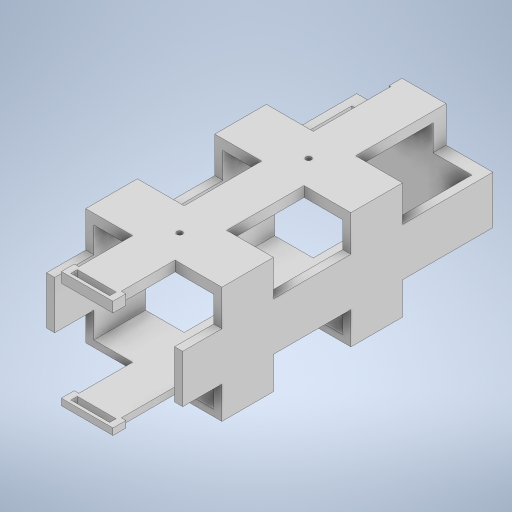
# Autodesk Inventor part: battery holder v2
Saved by Autodesk Inventor 2023 (Build 270158000, 158)
## iProperties
Created: 2023-01-11
Part Number: battery holder v2
Material: Generic
Document SubType Name: Modeling
Designer: agent
Density: 1 g/cm^3
Appearance: Default
Author: agent
Autodesk Inventor part; units mm, degrees
ref_plane "YZ Plane" through (0, 0, 0) normal (1, 0, 0) x (0, 1, 0)
ref_plane "XZ Plane" through (0, 0, 0) normal (0, 1, 0) x (-1, 0, 0)
ref_plane "XY Plane" through (0, 0, 0) normal (0, 0, 1) x (1, 0, 0)
sketch "Sketch1" plane through (0, 0, 0) normal (0, 1, 0) x (-1, 0, 0)
  line L0 (125.7746, -116.0471) -> (66.7746, -116.0471)
  line L1 (66.7746, -116.0471) -> (66.7746, 37.4129)
  line L2 (66.7746, 37.4129) -> (125.7746, 37.4129)
  line L3 (125.7746, 37.4129) -> (125.7746, -116.0471)
  point P0 (0, 0)
  dimension "d0" = 59
  dimension "d1" = 153.46
  constraints: 8 end point, 2 parallel, 1 horizontal, 1 perpendicular
  measures "d0" distance of L1.end L2.end
  measures "d1" distance between parallel lines of L2 L0
extrude "Extrusion1" add sketch "Sketch1" along normal blind 49
sketch "Sketch2" plane through (0, 0, 0) normal (0, -1, 0) x (1, 0, 0)
  line L0 (-125.7746, 37.4129) -> (-66.7746, 37.4129) projected
  line L1 (-66.7746, -116.0471) -> (-125.7746, -116.0471) projected
  line L2 (-85.8246, 37.4129) -> (-106.7246, 37.4129)
  line L3 (-106.7246, 37.4129) -> (-106.7246, -116.0471)
  line L4 (-106.7246, -116.0471) -> (-85.8246, -116.0471)
  line L5 (-85.8246, -116.0471) -> (-85.8246, 37.4129)
  line L6 (-66.7746, 37.4129) -> (-66.7746, -116.0471) projected
  line L7 (-125.7746, -116.0471) -> (-125.7746, 37.4129) projected
  point P0 (0, 0)
  dimension "d4" = 19.05
  dimension "d5" = 19.05
  constraints: 8 end point, 2 parallel, 2 point on line, 1 horizontal, 1 perpendicular
  measures "d4" distance between parallel lines of L6 L5
  measures "d5" distance between parallel lines of L7 L3
extrude "Extrusion2" add sketch "Sketch2" along normal blind 3.22 contours L0 L5 L1 L3
sketch "Sketch3" plane through (0, 49, 0) normal (0, 1, 0) x (1, 0, 0)
  line L0 (-125.7746, -37.4129) -> (-66.7746, -37.4129) projected
  line L1 (-106.7246, 116.0471) -> (-125.7746, 116.0471) projected
  line L2 (-85.8246, -37.4129) -> (-106.7246, -37.4129)
  line L3 (-106.7246, -37.4129) -> (-106.7246, 116.0471)
  line L4 (-106.7246, 116.0471) -> (-85.8246, 116.0471)
  line L5 (-85.8246, 116.0471) -> (-85.8246, -37.4129)
  line L6 (-66.7746, -37.4129) -> (-66.7746, 116.0471) projected
  line L7 (-125.7746, 116.0471) -> (-125.7746, -37.4129) projected
  point P0 (0, 0)
  dimension "d8" = 19.05
  dimension "d9" = 19.05
  constraints: 8 end point, 2 parallel, 2 point on line, 1 horizontal, 1 perpendicular
  measures "d8" distance between parallel lines of L6 L5
  measures "d9" distance between parallel lines of L7 L3
extrude "Extrusion3" add sketch "Sketch3" along normal blind 5 contours L3 L4 L5 L0
sketch "Sketch4" plane through (-66.7746, 0, 37.4129) normal (1, 0, 0) x (0, 0, -1)
  line L0 (0, 0) -> (0, 49) projected
  line L1 (153.46, 0) -> (153.46, 49) projected
  line L2 (0, 36.3) -> (153.46, 36.3)
  line L3 (153.46, 36.3) -> (153.46, 12.7)
  line L4 (153.46, 12.7) -> (0, 12.7)
  line L5 (0, 12.7) -> (0, 36.3)
  line L6 (0, 49) -> (153.46, 49) projected
  line L7 (0, 0) -> (153.46, 0) projected
  point P0 (37.4129, 0)
  point P1 (0, 12.7)
  dimension "d12" = 12.7
  dimension "d13" = 12.7
  constraints: 8 end point, 2 parallel, 2 point on line, 1 horizontal, 1 perpendicular
  measures "d12" distance between parallel lines of L6 L2
  measures "d13" distance between parallel lines of L7 L4
extrude "Extrusion4" add sketch "Sketch4" along normal blind 4 contours L0 L2 L1 L4
sketch "Sketch5" plane through (-125.7746, 0, -116.0471) normal (-1, 0, 0) x (0, 0, 1)
  line L0 (153.46, 0) -> (153.46, 49) projected
  line L1 (0, 0) -> (0, 49) projected
  line L2 (153.46, 12.7) -> (0, 12.7)
  line L3 (0, 12.7) -> (0, 36.3)
  line L4 (0, 36.3) -> (153.46, 36.3)
  line L5 (153.46, 36.3) -> (153.46, 12.7)
  line L6 (0, 0) -> (153.46, 0) projected
  line L7 (0, 49) -> (153.46, 49) projected
  point P0 (116.0471, 0)
  point P1 (0, 12.7)
  dimension "d16" = 12.7
  dimension "d17" = 12.7
  constraints: 8 end point, 2 parallel, 2 point on line, 1 horizontal, 1 perpendicular
  measures "d16" distance between parallel lines of L6 L2
  measures "d17" distance between parallel lines of L7 L4
extrude "Extrusion5" add sketch "Sketch5" along normal blind 4 contours L2 L1 L4 L0
sketch "Sketch6" plane through (-66.7746, 0, -116.0471) normal (0, 0, -1) x (-1, 0, 0)
  line L0 (63, -3.22) -> (-4, -3.22)
  line L1 (-4, -3.22) -> (-4, 54)
  line L2 (-4, 54) -> (63, 54)
  line L3 (63, 54) -> (63, -3.22)
  line L4 (19.05, 54) -> (39.95, 54) projected
  line L5 (63, 36.3) -> (63, 12.7) projected
  line L6 (-4, 12.7) -> (-4, 36.3) projected
  point P0 (-66.7746, 0)
  dimension "d20" = 0
  dimension "d21" = 0
  dimension "d22" = 0
  constraints: 8 end point, 2 parallel, 1 horizontal, 1 perpendicular
  measures "d20" distance between parallel lines of L4 L2
  measures "d21" distance between parallel lines of L5 L3
  measures "d22" distance between parallel lines of L6 L1
extrude "Extrusion6" add sketch "Sketch6" along normal blind 6.395
sketch "Sketch7" plane through (-129.7746, 0, -116.0471) normal (-1, 0, 0) x (0, 0, 1)
  line L0 (153.46, 54) -> (0, 54) projected
  line L1 (153.46, -3.22) -> (0, -3.22) projected
  line L2 (38.1, 54) -> (63.5, 54)
  line L3 (63.5, 54) -> (63.5, -3.22)
  line L4 (63.5, -3.22) -> (38.1, -3.22)
  line L5 (38.1, -3.22) -> (38.1, 54)
  line L6 (101.6, 54) -> (127, 54)
  line L7 (127, 54) -> (127, -3.22)
  line L8 (127, -3.22) -> (101.6, -3.22)
  line L9 (101.6, -3.22) -> (101.6, 54)
  line L10 (0, 36.3) -> (0, 54) projected
  point P0 (116.0471, 0)
  point P1 (127, -3.22)
  dimension "d25" = 38.1
  dimension "d26" = 38.1
  dimension "d27" = 25.4
  dimension "d28" = 25.4
  constraints: 16 end point, 4 parallel, 4 point on line, 2 horizontal, 2 perpendicular
  measures "d25" distance between parallel lines of L10 L5
  measures "d26" distance between parallel lines of L9 L3
  measures "d27" distance between parallel lines of L3 L5
  measures "d28" distance between parallel lines of L7 L9
extrude "Extrusion7" add sketch "Sketch7" against normal up to surface (67 mm away) contours L7 L1 L9 L0 | L3 L1 L5 L0
sketch "Sketch8" plane through (-125.7746, 0, 37.4129) normal (0, 0, 1) x (1, 0, 0)
  line L0 (39.95, 49) -> (59, 49) projected
  line L1 (-4, 54) -> (19.05, 54) projected
  line L2 (42.2021, 49) -> (16.8021, 49)
  line L3 (16.8021, 49) -> (16.8021, 54)
  line L4 (16.8021, 54) -> (42.2021, 54)
  line L5 (42.2021, 54) -> (42.2021, 49)
  line L6 (19.05, 49) -> (19.05, 54) projected
  line L7 (0, 0) -> (19.05, 0) projected
  line L8 (39.95, -3.22) -> (63, -3.22) projected
  line L9 (16.8021, 0) -> (42.2021, 0)
  line L10 (42.2021, 0) -> (42.2021, -3.22)
  line L11 (42.2021, -3.22) -> (16.8021, -3.22)
  line L12 (16.8021, -3.22) -> (16.8021, 0)
  point P0 (125.7746, 0)
  point P1 (42.2021, 51.5)
  point P2 (16.8021, 51.5)
  point P3 (19.05, 51.5)
  dimension "d31" = 25.4
  dimension "d32" = 2.2479
  constraints: 16 end point, 4 parallel, 4 point on line, 3 midpoint, 2 horizontal, 2 perpendicular
  measures "d31" distance of point (42.202, 51.5) point (16.802, 51.5)
  measures "d32" distance of point (16.802, 51.5) point (19.05, 51.5)
extrude "Extrusion8" add sketch "Sketch8" along normal blind 6.35
sketch "Sketch9" plane through (0, 54, 0) normal (0, 1, 0) x (1, 0, 0)
  line L0 (-118.2456, -83.2824) -> (-137.2956, -83.2824)
  line L1 (-137.2956, -83.2824) -> (-137.2956, -80.1074)
  line L2 (-137.2956, -80.1074) -> (-118.2456, -80.1074)
  line L3 (-118.2456, -80.1074) -> (-118.2456, -83.2824)
  line L4 (-86.7475, -39.0639) -> (-105.7975, -39.0639)
  line L5 (-105.7975, -39.0639) -> (-105.7975, -42.2389)
  line L6 (-105.7975, -42.2389) -> (-86.7475, -42.2389)
  line L7 (-86.7475, -42.2389) -> (-86.7475, -39.0639)
  line L8 (-83.5725, -43.7629) -> (-108.9725, -43.7629) projected
  line L9 (-83.5725, -37.4129) -> (-83.5725, -43.7629) projected
  point P0 (0, 0)
  point P1 (-118.2456, -81.6949)
  point P2 (-137.2956, -81.6949)
  point P3 (-105.7975, -40.6514)
  point P4 (-86.7475, -40.6514)
  point P5 (-83.5725, -40.5879)
  dimension "d35" = 3.175
  dimension "d36" = 19.05
  dimension "d37" = 19.05
  dimension "d38" = 3.175
  dimension "d39" = 1.524
  dimension "d40" = 3.175
  constraints: 16 end point, 5 midpoint, 3 parallel, 1 horizontal, 1 perpendicular
  measures "d35" distance between parallel lines of L0 L2
  measures "d36" distance of point (-118.246, -81.695) point (-137.296, -81.695)
  measures "d37" distance from line of point (-105.797, -40.651) L7
  measures "d38" distance between parallel lines of L4 L6
  measures "d39" distance between parallel lines of L8 L6
  measures "d40" horizontal distance of point (-86.747, -40.651) point (-83.572, -40.588)
extrude "Extrusion9" cut sketch "Sketch9" against normal up to surface (57.22 mm away) contours L7 L6 L5 L4
sketch "Sketch10" plane through (-66.7746, 12.7, 37.4129) normal (0, 0, 1) x (1, 0, 0)
  line L0 (-59, 23.6) -> (-59, 36.3) projected
  line L1 (0, 0) -> (0, -12.7) projected
  line L2 (-59, 36.3) -> (0, 36.3)
  line L3 (0, 36.3) -> (0, -12.7)
  line L4 (0, -12.7) -> (-59, -12.7)
  line L5 (-59, -12.7) -> (-59, 36.3)
  point P0 (66.7746, -12.7)
  point P1 (-59, 23.6)
  constraints: 8 end point, 2 parallel, 1 horizontal, 1 perpendicular
extrude "Extrusion10" cut sketch "Sketch10" against normal up to surface (153.46 mm away)
sketch "Sketch11" plane through (0, 54, 0) normal (0, 1, 0) x (1, 0, 0)
  line L0 (-85.8246, 116.0471) -> (-85.8246, 77.9471) projected
  line L1 (-129.7746, 52.5471) -> (-106.7246, 52.5471) projected
  line L2 (-85.8246, 52.5471) -> (-85.8246, 14.4471) projected
  line L3 (-129.7746, -10.9529) -> (-106.7246, -10.9529) projected
  circle A0 centre (-96.2746, 65.2471) radius 1.35
  circle A1 centre (-96.2746, 1.7471) radius 1.35
  point P0 (0, 0)
  dimension "d45" = 2.7
  dimension "d46" = 2.7
  dimension "d47" = 63.5
  constraints: 2 centre point
  measures "d45" diameter of A0
  measures "d46" diameter of A1
  measures "d47" distance of A1.centre A0.centre
extrude "Extrusion11" cut sketch "Sketch11" against normal up to surface (57.22 mm away)
sketch "Sketch12" plane through (-108.9725, 49, 43.7629) normal (0, -1, 0) x (1, 0, 0)
  circle A0 centre (12.6979, -45.51) radius 1.35 projected
  circle A1 centre (12.6979, -45.51) radius 3.175
  circle A2 centre (12.6979, -109.01) radius 1.35 projected
  circle A3 centre (12.6979, -109.01) radius 3.175
  point P0 (108.9725, -43.7629)
  dimension "d50" = 6.35
  dimension "d51" = 6.35
  constraints: 2 centre point, 2 coincident
  measures "d50" diameter of A1
  measures "d51" diameter of A3
extrude "Extrusion12" cut sketch "Sketch12" against normal blind 2 contours A0 | A1 | A2 | A3
sketch "Sketch13" plane through (-129.7746, 0, -116.0471) normal (-1, 0, 0) x (0, 0, 1)
  line L0 (153.46, 36.3) -> (127, 36.3) projected
  line L1 (127, 12.7) -> (153.46, 12.7) projected
  line L2 (153.46, 36.3) -> (146.2804, 36.3)
  line L3 (146.2804, 36.3) -> (146.2804, 12.7)
  line L4 (146.2804, 12.7) -> (153.46, 12.7)
  line L5 (153.46, 12.7) -> (153.46, 36.3)
  point P0 (116.0471, 0)
  constraints: 8 end point, 2 parallel, 1 horizontal, 1 perpendicular, 1 point on line
extrude "Extrusion13" cut sketch "Sketch13" against normal up to surface (67 mm away)
sketch "Sketch14" plane through (-66.7746, 0, -122.4421) normal (0, 0, -1) x (-1, 0, 0)
  line L0 (-4, 36.3) -> (-4, 54) projected
  line L1 (-4, 54) -> (19.05, 54)
  line L2 (19.05, 54) -> (19.05, 36.3)
  line L3 (19.05, 36.3) -> (-4, 36.3)
  line L4 (-4, 36.3) -> (-4, 54)
  line L5 (63, -3.22) -> (63, 54) projected
  line L6 (63, 54) -> (40.73, 54)
  line L7 (40.73, 54) -> (40.73, 36.3)
  line L8 (40.73, 36.3) -> (63, 36.3)
  line L9 (63, 36.3) -> (63, 54)
  line L10 (63, 12.7) -> (63, -3.22) projected
  line L11 (63, -3.22) -> (39.95, -3.22) projected
  line L12 (63, 12.7) -> (39.95, 12.7)
  line L13 (39.95, 12.7) -> (39.95, -3.22)
  line L14 (39.95, -3.22) -> (63, -3.22)
  line L15 (63, -3.22) -> (63, 12.7)
  line L16 (-4, 12.7) -> (-4, -3.22) projected
  line L17 (-4, -3.22) -> (19.05, -3.22)
  line L18 (19.05, -3.22) -> (19.05, 12.7)
  line L19 (19.05, 12.7) -> (-4, 12.7)
  line L20 (-4, 12.7) -> (-4, -3.22)
  point P0 (-66.7746, 0)
  point P1 (19.05, 54)
  point P2 (-4, 12.7)
  point P3 (63, 36.3)
  point P4 (63, 36.3)
  dimension "d56" = 0
  dimension "d59" = 0
  dimension "d60" = 0
  constraints: 32 end point, 8 parallel, 4 horizontal, 4 perpendicular, 1 point on line
  measures "d56" distance from line of point (19.05, 54) L2
  measures "d59" distance from line of point (63, 36.3) L8
  measures "d60" distance from line of L0.start L3
extrude "Extrusion14" cut sketch "Sketch14" against normal up to surface (6.395 mm away)
body "Solid1"
